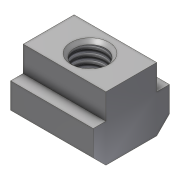
# Autodesk Inventor part: T-Nutenstein 8 - M6
Saved by Autodesk Inventor 2015 (Build 190159000, 159)
## iProperties
Created: 2012-06-24
Part Number: T-Nutenstein 8 - M6
Material: Steel
Document SubType Name: Modeling
Density: 7.85 g/cm^3
Appearance: Steel
Autodesk Inventor part; units mm, degrees
ref_plane "YZ Plane" through (0, 0, 0) normal (1, 0, 0) x (0, 1, 0)
ref_plane "XZ Plane" through (0, 0, 0) normal (0, 1, 0) x (-1, 0, 0)
ref_plane "XY Plane" through (0, 0, 0) normal (0, 0, 1) x (1, 0, 0)
sketch "Sketch1" plane through (0, 0, 0) normal (1, 0, 0) x (0, 1, 0)
  line L0 (0, 0) -> (4, 0)
  line L1 (4, 0) -> (6, 2)
  line L2 (6, 2) -> (6, 6)
  line L3 (6, 6) -> (4, 6)
  line L4 (4, 6) -> (4, 10)
  line L5 (4, 10) -> (0, 10)
  line L6 (0, -2) -> (0, 12) projected
  line L7 (0, 0) -> (-4, 0)
  line L8 (-4, 0) -> (-6, 2)
  line L9 (-6, 2) -> (-6, 6)
  line L10 (-6, 6) -> (-4, 6)
  line L11 (-4, 6) -> (-4, 10)
  line L12 (-4, 10) -> (0, 10)
  dimension "d0" = 10
  dimension "d1" = 45
  dimension "d4" = 2
  dimension "d6" = 6
  dimension "d19" = 12
  dimension "d20" = 8
  constraints: 24 end point, 5 symmetric about line, 3 parallel, 2 perpendicular, 1 horizontal, 1 point on line
  measures "d0" distance between parallel lines of L0 L5
  measures "d1" angle of L0 L1
  measures "d4" distance from line of L1.end L0
  measures "d6" distance between parallel lines of L0 L3
  measures "d19" diameter of L2 L6
  measures "d20" diameter of L4 L6
extrude "Extrusion1" add sketch "Sketch1" along normal mid plane 13
sketch "Sketch2" plane through (6.5, -4, 10) normal (0, 0, 1) x (0, 1, 0)
  point P0 (4, 6.5)
hole "Hole1" at (0, 0, 10) direction (0, 0, -1) diameter 4.917 end through all thread size "M6x1" class "6H" standard "ISO Metric profile"
chamfer "Chamfer1" distance 0.5415 angle 45 2 edges at (0, 2.4585, 10) (0, 2.4585, 0)
body "Solid1"
